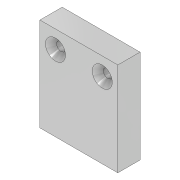
# Autodesk Inventor part: Soporte para Patas Regulables
Saved by Autodesk Inventor 2020 (Build 240168000, 168)
## iProperties
Created: 2020-05-22
Part Number: Soporte para Patas Regulables
Material: Aluminum 6061
Document SubType Name: Modeling
Designer: Dante
Density: 2.7 g/cm^3
Appearance: Aluminum - Dark
Mass: 58.5912 g
Surface Area: 74.4655 cm^2
Volume: 21.7004 cm^3
Author: Dante
Autodesk Inventor part; units mm, degrees
ref_plane "YZ Plane" through (0, 0, 0) normal (1, 0, 0) x (0, 1, 0)
ref_plane "XZ Plane" through (0, 0, 0) normal (0, 1, 0) x (-1, 0, 0)
ref_plane "XY Plane" through (0, 0, 0) normal (0, 0, 1) x (1, 0, 0)
sketch "Sketch1" plane through (0, 0, 0) normal (0, 0, 1) x (1, 0, 0)
  line L0 (-5, -18.8059) -> (-5, -60.8059)
  line L1 (-5, -60.8059) -> (30, -60.8059)
  line L2 (30, -60.8059) -> (30, -18.8059)
  circle A0 centre (2, -26.8059) radius 2
  circle A1 centre (23, -26.8059) radius 2
  circle A2 centre (2, -26.8059) radius 4
  circle A3 centre (23, -26.8059) radius 4
  line L3 (30, -18.8059) -> (-5, -18.8059)
  point P0 (0, -10)
  dimension "d17" = 35
  dimension "d19" = 4
  dimension "d20" = 4
  dimension "d22" = 8
  dimension "d23" = 8
  dimension "d29" = 7
  dimension "d60" = 42
  dimension "d61" = 8
  dimension "d62" = 8
  dimension "d63" = 21
  constraints: 8 end point, 4 centre point, 2 coincident, 2 perpendicular, 1 horizontal, 1 vertical
  measures "d17" distance of L0.end L1.end
  measures "d19" diameter of A0
  measures "d20" diameter of A1
  measures "d22" diameter of A2
  measures "d23" diameter of A3
  measures "d29" distance from line of L2 A1.centre
  measures "d60" distance between parallel lines of L1 L3
  measures "d61" distance from line of L3 A0.centre
  measures "d62" distance from line of L3 A1.centre
  measures "d63" distance of A0.centre A1.centre
extrude "Extrusion2" add sketch "Sketch1" along normal blind 10 contours L3 L2 L1 L0 | A2 | A3
sketch "Sketch4" plane through (-5, -60.8059, 0) normal (0, -1, 0) x (1, 0, 0)
  circle A0 centre (17.5, 5) radius 3
  line L0 (35, 0) -> (35, 10) projected
  line L1 (0, 10) -> (35, 10) projected
  dimension "d48" = 6
  dimension "d49" = 17.5
  dimension "d50" = 5
  constraints: 1 centre point
  measures "d48" diameter of A0
  measures "d49" distance from line of A0.centre L0
  measures "d50" distance from line of L1 A0.centre
extrude "Extrusion5" cut sketch "Sketch4" against normal blind 30
thread "Thread2" size "M6x1" class "6H" standard "ANSI Metric M Profile" length 25
chamfer "Chaflán1" distance 2.5 angle 45 2 edges at (0, -26.8059, 10) (21, -26.8059, 10)
equation "\"d61\" = d62"
body "Solid2"
